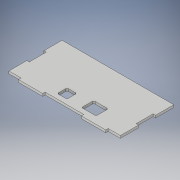
# Autodesk Inventor part: Part Sisi 3
Saved by Autodesk Inventor 2019 (Build 230136000, 136)
## iProperties
Created: 2019-07-08
Part Number: Part Sisi 3
Material: Generic
Document SubType Name: Modeling
Designer: azriel
Density: 1 g/cm^3
Appearance: Default
Author: azriel
Autodesk Inventor part; units mm, degrees
ref_plane "YZ Plane" through (0, 0, 0) normal (1, 0, 0) x (0, 1, 0)
ref_plane "XZ Plane" through (0, 0, 0) normal (0, 1, 0) x (-1, 0, 0)
ref_plane "XY Plane" through (0, 0, 0) normal (0, 0, 1) x (1, 0, 0)
sketch "Sketch1" plane through (0, 0, 0) normal (0, 1, 0) x (-1, 0, 0)
  line L0 (47.6597, 73.3148) -> (47.6597, 78.3148)
  line L1 (97.6593, 78.3148) -> (97.6593, 72.863)
  line L2 (-82.3403, 73.3148) -> (-82.3403, 78.3148)
  line L3 (-32.3403, 78.3148) -> (-32.3403, 73.3148)
  line L4 (117.6597, 72.863) -> (97.6593, 72.863)
  line L5 (47.6597, 73.3148) -> (-32.3403, 73.3148)
  line L6 (-82.3403, 73.3148) -> (-107.3403, 73.3148)
  line L7 (-20.3403, 63.3147) -> (-44.3403, 63.3147)
  line L8 (-47.3403, 60.3147) -> (-47.3403, 41.3147)
  line L9 (-44.3403, 38.3147) -> (-20.3403, 38.3147)
  line L10 (-17.3403, 41.3147) -> (-17.3403, 60.3147)
  line L11 (29.6597, 63.3147) -> (15.6597, 63.3147)
  line L12 (12.6597, 60.3147) -> (12.6597, 46.3147)
  line L13 (15.6597, 43.3147) -> (29.6597, 43.3147)
  line L14 (32.6597, 46.3147) -> (32.6597, 60.3147)
  arc A0 (29.6597, 43.3147) -> (32.6597, 46.3147) centre (29.6597, 46.3147) ccw
  arc A1 (32.6597, 60.3147) -> (29.6597, 63.3147) centre (29.6597, 60.3147) ccw
  arc A2 (15.6597, 63.3147) -> (12.6597, 60.3147) centre (15.6597, 60.3147) ccw
  arc A3 (12.6597, 46.3147) -> (15.6597, 43.3147) centre (15.6597, 46.3147) ccw
  arc A4 (-20.3403, 38.3147) -> (-17.3403, 41.3147) centre (-20.3403, 41.3147) ccw
  arc A5 (-47.3403, 41.3147) -> (-44.3403, 38.3147) centre (-44.3403, 41.3147) ccw
  arc A6 (-44.3403, 63.3147) -> (-47.3403, 60.3147) centre (-44.3403, 60.3147) ccw
  arc A7 (-17.3403, 60.3147) -> (-20.3403, 63.3147) centre (-20.3403, 60.3147) ccw
  line L15 (97.6597, -36.6853) -> (117.6597, -36.6853)
  line L16 (-107.3403, -36.6853) -> (-82.3403, -36.6853)
  line L17 (-32.3403, -36.6853) -> (47.6597, -36.6853)
  line L18 (-107.3403, 0.8147) -> (-107.3403, -36.6853)
  line L19 (-107.3403, 0.8147) -> (-102.3403, 0.8147)
  line L20 (-102.3403, 0.8147) -> (-102.3403, 35.8147)
  line L21 (-102.3403, 35.8147) -> (-107.3403, 35.8147)
  line L22 (-107.3403, 35.8147) -> (-107.3403, 73.3148)
  line L23 (117.6597, -36.6853) -> (122.6597, -36.6853)
  line L24 (122.6597, -36.6853) -> (122.6597, 0.8147)
  line L25 (122.6597, 0.8147) -> (117.6597, 0.8147)
  line L26 (117.6597, 0.8147) -> (117.6597, 35.8147)
  line L27 (122.6902, 35.8147) -> (122.6902, 72.863)
  line L28 (122.6902, 72.863) -> (117.6597, 72.863)
  line L29 (122.6902, 35.8147) -> (117.6597, 35.8147)
  line L30 (97.6597, -36.6853) -> (-82.3403, -36.6853)
  line L31 (-32.3403, 73.3148) -> (-32.3403, 78.3148)
  line L32 (-32.3403, 78.3148) -> (-82.3403, 78.3148)
  line L33 (47.6597, 78.3148) -> (97.6593, 78.3148)
  point P0 (-17.3403, 63.3147)
  point P1 (-47.3403, 63.3147)
  point P2 (-47.3403, 38.3147)
  point P3 (32.6597, 63.3147)
  point P4 (12.6597, 63.3147)
  point P5 (12.6597, 43.3147)
  dimension "d4" = 80
  dimension "d19" = 30
  dimension "d20" = 25
  dimension "d28" = 20
  dimension "d29" = 20
  dimension "d30" = 30
  dimension "d31" = 3
  dimension "d41" = 5
  dimension "d53" = 5
  constraints: 68 end point, 16 parallel, 16 point on circle, 16 tangent, 14 point on line, 10 perpendicular, 8 centre point, 7 equal radius, 5 horizontal, 1 vertical
  measures "d4" distance between parallel lines of L0 L3
  measures "d19" distance of point (-17.34, 63.315) point (-47.34, 63.315)
  measures "d20" distance of point (-47.34, 38.315) point (-47.34, 63.315)
  measures "d28" distance of point (32.66, 63.315) point (12.66, 63.315)
  measures "d29" distance of point (12.66, 43.315) point (12.66, 63.315)
  measures "d30" distance between parallel lines of L10 L12
  measures "d31" radius of A0
  measures "d41" distance of L18.start L19.end
  measures "d53" distance of L3.start L3.end
extrude "Extrusion3" add sketch "Sketch1" along normal blind 5
body "Solid3"
